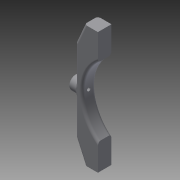
# Autodesk Inventor part: Stuetze
Saved by Autodesk Inventor 2015 SP2 (Build 190223200, 223)
## iProperties
Created: 2024-01-04
Part Number: Stuetze
Material: Generisch
Document SubType Name: Modeling
Designer: montag01
Density: 1 g/cm^3
Appearance: Vorgabe
Author: montag01
Autodesk Inventor part; units mm, degrees
ref_plane "YZ Plane" through (0, 0, 0) normal (1, 0, 0) x (0, 1, 0)
ref_plane "XZ Plane" through (0, 0, 0) normal (0, 1, 0) x (-1, 0, 0)
ref_plane "XY Plane" through (0, 0, 0) normal (0, 0, 1) x (1, 0, 0)
sketch "Skizze1" plane through (0, 0, 0) normal (0, 1, 0) x (-1, 0, 0)
  line L0 (0, 0) -> (0, -30)
  line L1 (-16.6, -44.8) -> (-6.6, -44.8)
  line L2 (-6.6, -44.8) -> (0, -30)
  line L3 (0, 0) -> (0, 30)
  line L4 (-16.6, 44.8) -> (-6.6, 44.8)
  line L5 (-6.6, 44.8) -> (0, 30)
  arc A0 (-16.6, -25.2354) -> (-16.6, 25.2354) centre (-38, 0) ccw
  line L6 (-16.6, -44.8) -> (-16.6, -25.2354)
  line L7 (-16.6, 44.8) -> (-16.6, 25.2354)
  dimension "d0" = 30
  dimension "d6" = 10
  constraints: 16 end point, 3 vertical, 2 point on circle, 1 centre point
  measures "d0" distance of L0.start L0.end
  measures "d6" distance of L1.start L1.end
extrude "Extrusion1" add sketch "Skizze1" along normal blind 10
sketch "Skizze2" plane through (0, 0, -30) normal (-1, 0, 0) x (0, 0, 1)
  circle A0 centre (30, 5) radius 5
  point P0 (30, 0)
  dimension "d13" = 10
  constraints: 1 centre point
  measures "d13" diameter of A0
extrude "Extrusion2" add sketch "Skizze2" along normal blind 5
fillet "Rundung1" radius 2 1 edges at (0, 5, -30)
fillet "Rundung2" radius 2 1 edges at (0, 5, 30)
fillet "Rundung3" radius 2 12 edges at (3.3867, 10, 37.5944) (0.0438, 10, 29.9907) (0, 10, 14.7871) (0.0438, 0, 29.9907) (0, 0, 14.7871) (3.3867, 0, 37.5944) (0.0438, 10, -29.9907) (3.3867, 10, -37.5944) (0, 10, -14.7871) (0.0438, 0, -29.9907) (3.3867, 0, -37.5944) (0, 0, -14.7871)
fillet "Rundung4" radius 1 1 edges at (-5, 5, -5)
fillet "Rundung5" radius 2 2 edges at (4.9125, 10, 0) (4.9125, 0, 0)
sketch "Skizze3" plane through (-5, 5, 0) normal (-1, 0, 0) x (0, 0, 1)
  circle A0 centre (0, 0) radius 1.25
  point P0 (0, -5)
  dimension "d21" = 2.5
  constraints: 1 centre point
  measures "d21" diameter of A0
extrude "Extrusion3" cut sketch "Skizze3" against normal blind 10
